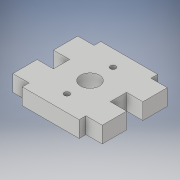
# Autodesk Inventor part: thumper-bumper-top-v3
Saved by Autodesk Inventor 2017 (Build 210142000, 142)
## iProperties
Created: 2017-02-22
Part Number: thumper-bumper-top-v3
Material: Generic
Document SubType Name: Modeling
Designer: John
Density: 1 g/cm^3
Appearance: Default
Author: John
Autodesk Inventor part; units mm, degrees
ref_plane "YZ Plane" through (0, 0, 0) normal (1, 0, 0) x (0, 1, 0)
ref_plane "XZ Plane" through (0, 0, 0) normal (0, 1, 0) x (-1, 0, 0)
ref_plane "XY Plane" through (0, 0, 0) normal (0, 0, 1) x (1, 0, 0)
sketch "Sketch1" plane through (0, 0, 0) normal (0, 1, 0) x (-1, 0, 0)
  line L0 (1.2471, 10.6093) -> (-19.7529, 10.6093)
  line L1 (-19.7529, 10.6093) -> (-19.7529, -18.3907)
  line L2 (-19.7529, -18.3907) -> (1.2471, -18.3907)
  line L3 (1.2471, -15.8907) -> (7.2471, -15.8907)
  line L4 (7.2471, -15.8907) -> (7.2471, -6.8907)
  line L5 (7.2471, -6.8907) -> (1.2471, -6.8907)
  line L6 (1.2471, -6.8907) -> (1.2471, -15.8907)
  line L7 (1.2471, -3.8907) -> (-9.2529, -3.8907) construction
  line L8 (-9.2529, -18.3907) -> (-9.2529, 10.6093) construction
  line L9 (1.2471, 8.1093) -> (7.2471, 8.1093)
  line L10 (7.2471, 8.1093) -> (7.2471, -0.8907)
  line L11 (7.2471, -0.8907) -> (1.2471, -0.8907)
  line L12 (1.2471, -0.8907) -> (1.2471, 8.1093)
  line L13 (-19.7529, -15.8907) -> (-25.7529, -15.8907)
  line L14 (-25.7529, -15.8907) -> (-25.7529, -6.8907)
  line L15 (-25.7529, -6.8907) -> (-19.7529, -6.8907)
  line L16 (-19.7529, -6.8907) -> (-19.7529, -15.8907)
  line L17 (-19.7529, 8.1093) -> (-25.7529, 8.1093)
  line L18 (-25.7529, 8.1093) -> (-25.7529, -0.8907)
  line L19 (-25.7529, -0.8907) -> (-19.7529, -0.8907)
  line L20 (-19.7529, -0.8907) -> (-19.7529, 8.1093)
  line L21 (1.2471, -15.8907) -> (1.2471, 8.1093)
  line L22 (-9.2529, -3.8907) -> (-19.7529, -3.8907) construction
  line L23 (1.2471, -18.3907) -> (1.2471, 10.6093)
  dimension "d49" = 21
  dimension "d50" = 29
  dimension "d54" = 9
  dimension "d60" = 6
  dimension "d76" = 6
  constraints: 48 end point, 12 symmetric about line, 6 parallel, 4 midpoint, 3 collinear, 2 horizontal, 2 perpendicular
  measures "d49" distance of L2.end L1.end
  measures "d50" distance of L1.end L0.end
  measures "d54" distance of L4.end L3.end
  measures "d60" distance between parallel lines of L5 L11
  measures "d76" distance between parallel lines of L21 L4
extrude "Extrusion1" add sketch "Sketch1" along normal blind 6
sketch "Sketch3" plane through (0, 6, 0) normal (0, 1, 0) x (1, 0, 0)
  line L0 (19.7529, 18.3907) -> (-1.2471, 18.3907) construction
  line L1 (9.2529, 18.3907) -> (9.2529, -10.6093) construction
  line L2 (-1.2471, -10.6093) -> (19.7529, -10.6093) construction
  line L3 (-1.2471, 0.8907) -> (-1.2471, 6.8907) construction
  line L4 (-1.2471, 3.8907) -> (19.7529, 3.8907) construction
  line L5 (19.7529, 0.8907) -> (19.7529, 6.8907) construction
  circle A0 centre (9.2529, 12.3907) radius 1
  circle A1 centre (9.2529, -4.6093) radius 1
  circle A2 centre (9.2529, 3.8907) radius 3.5
  point P0 (0, 0)
  dimension "d91" = 2
  dimension "d92" = 8.5
  dimension "d96" = 7
  constraints: 5 midpoint, 4 end point, 3 centre point, 1 point on line, 1 symmetric about line, 1 other
  measures "d91" diameter of A0
  measures "d92" distance from line of L4 A0.centre
  measures "d96" diameter of A2
extrude "Extrusion3" cut sketch "Sketch3" against normal through all
body "Solid1"
